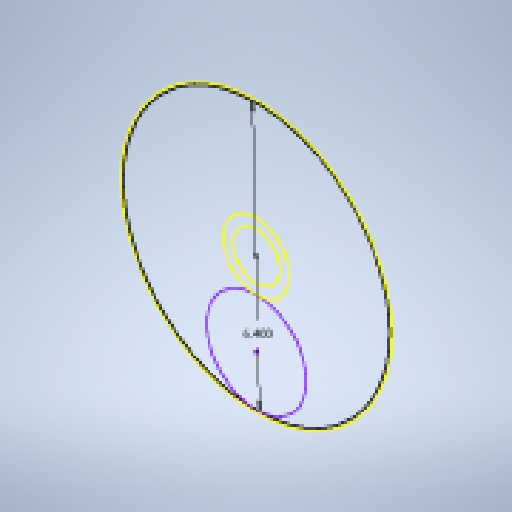
# Autodesk Inventor part: GearsTest2
Saved by Autodesk Inventor 2023 (Build 270158030, 158C)
## iProperties
Created: 2024-09-26
Part Number: GearsTest2
Material: Generic
Document SubType Name: Modeling
Designer: lvrectanus0
Density: 1 g/cm^3
Appearance: Default
Author: lvrectanus0
Autodesk Inventor part; units mm, degrees
ref_plane "YZ Plane" through (0, 0, 0) normal (1, 0, 0) x (0, 1, 0)
ref_plane "XZ Plane" through (0, 0, 0) normal (0, 1, 0) x (-1, 0, 0)
sketch "Sketch1" plane through (0, 0, 0) normal (0, 0, 1) x (1, 0, 0)
  circle A0 centre (0, 0) radius 14.351 projected
  circle A1 centre (0, 0) radius 82.55 projected
  circle A2 centre (0, 0) radius 81.28
  circle A3 centre (0, -51.435) radius 29.845
  circle A4 centre (0, -51.435) radius 34.925
  circle A5 centre (0, 0) radius 21.59 projected
  point P0 (-22.577, -78.0815)
  point P1 (0, -81.28)
  point P2 (22.577, -78.0815)
  dimension "d0" = 162.56
  dimension "d3" = 5.08
  constraints: 3 centre point, 2 coincident, 2 tangent
  measures "d0" diameter of A2
  measures "d3" radial gap between concentric circles of A4 A3
ref_plane "Work Plane1" through (-15.4305, -15.4305, 1.524) normal (0, 0, 1) x (1, 0, 0)
extrude "Extrusion1" add sketch "Sketch1" along normal up to surface (1.524 mm away) contours A4 A5 A3 A2 | A2 A3 A5 A4 | A3 | A4 A5 picked at (0, -18.3438)
body "Solid1"
